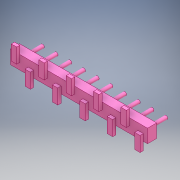
# Autodesk Inventor part: Circuit_PSM-410233-00
Saved by Autodesk Inventor 2018 (Build 220112000, 112)
## iProperties
Created: 2018-02-16
Part Number: Circuit_PSM-410233-00
Material: 一般
Document SubType Name: Modeling
Designer: sktom
Density: 1 g/cm^3
Appearance: ピンク
Author: sktom
Autodesk Inventor part; units mm, degrees
ref_plane "YZ Plane" through (0, 0, 0) normal (1, 0, 0) x (0, 1, 0)
ref_plane "XZ Plane" through (0, 0, 0) normal (0, 1, 0) x (-1, 0, 0)
ref_plane "XY Plane" through (0, 0, 0) normal (0, 0, 1) x (1, 0, 0)
sketch "スケッチ1" plane through (0, 0, 0) normal (0, 0, 1) x (1, 0, 0)
  line L0 (-1.27, 1.15) -> (1.27, 1.15)
  line L1 (1.27, 1.15) -> (1.27, -1.15)
  line L2 (1.27, -1.15) -> (-1.27, -1.15)
  line L3 (-1.27, -1.15) -> (-1.27, 1.15)
  line L4 (-1.27, 1.15) -> (1.27, -1.15) construction
  line L5 (1.27, 1.15) -> (-1.27, -1.15) construction
  point P0 (0, 0)
  dimension "d0" = 2.54
  dimension "d1" = 2.3
  constraints: 12 end point, 2 midpoint, 2 parallel, 1 horizontal, 1 perpendicular
  measures "d0" distance of L0.start L0.end
  measures "d1" distance of L0.end L1.end
extrude "押し出し1" add sketch "スケッチ1" along normal blind 2.5
sketch "スケッチ2" plane through (-1.27, 1.15, 0) normal (0, 1, 0) x (1, 0, 0)
  circle A0 centre (1.27, -1.25) radius 0.32
  line L0 (0, 0) -> (2.54, 0) projected
  line L1 (0, 0) -> (0, -2.5) projected
  point P0 (1.27, 0)
  point P1 (1.27, 0)
  point P2 (0, -1.25)
  dimension "d4" = 0.64
  constraints: 2 midpoint, 1 centre point, 1 horizontal alignment, 1 vertical alignment
  measures "d4" diameter of A0
extrude "押し出し2" add sketch "スケッチ2" along normal blind 3
pattern_linear "矩形状パターン1" count 2 spacing 2.54 along (1, 0, 0) of "押し出し2", "押し出し1"
sketch "スケッチ3" plane through (-1.27, -1.15, 0) normal (0, -1, 0) x (1, 0, 0)
  line L0 (0.77, 1.25) -> (1.77, 1.25)
  line L1 (1.77, 1.25) -> (1.77, 4)
  line L2 (1.77, 4) -> (0.77, 4)
  line L3 (0.77, 4) -> (0.77, 1.25)
  line L4 (3.31, 1.25) -> (4.31, 1.25)
  line L5 (4.31, 1.25) -> (4.31, -1.5)
  line L6 (4.31, -1.5) -> (3.31, -1.5)
  line L7 (3.31, -1.5) -> (3.31, 1.25)
  line L8 (5.08, 0) -> (5.08, 2.5) projected
  circle A0 centre (1.27, 1.25) radius 0.32 construction
  circle A1 centre (3.81, 1.25) radius 0.32 construction
  point P0 (1.27, 0)
  point P1 (5.08, 1.25)
  dimension "d10" = 1
  dimension "d11" = 5.5
  constraints: 16 end point, 6 parallel, 3 midpoint, 2 coincident, 2 horizontal, 2 horizontal alignment, 2 perpendicular
  measures "d10" distance of L0.start L0.end
  measures "d11" distance between parallel lines of L6 L2
extrude "押し出し3" add sketch "スケッチ3" along normal blind 0.6
move faces "移動1" translate (0, 0.6, 0) faces at (-0.1667, -1.15, 3.5) (2.3733, -1.15, -0.5)
move faces "移動2" translate (0, 0.6, 0) faces at (0.4233, -1.15, 0.4167) (2.7067, -1.75, 0.3333) (0.1667, -1.75, 2.1667)
pattern_linear "矩形状パターン2" count 5 spacing 5.08 along (1, 0, 0)
